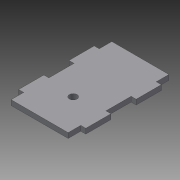
# Autodesk Inventor part: top
Saved by Autodesk Inventor 2015 (Build 190159000, 159)
## iProperties
Created: 2017-03-04
Part Number: top
Material: Generic
Document SubType Name: Modeling
Designer: Guy
Density: 1 g/cm^3
Appearance: Default
Author: Guy
Autodesk Inventor part; units mm, degrees
ref_plane "YZ Plane" through (0, 0, 0) normal (1, 0, 0) x (0, 1, 0)
ref_plane "XZ Plane" through (0, 0, 0) normal (0, 1, 0) x (-1, 0, 0)
ref_plane "XY Plane" through (0, 0, 0) normal (0, 0, 1) x (1, 0, 0)
sketch "Sketch1" plane through (0, 0, 0) normal (0, 0, 1) x (1, 0, 0)
  line L0 (0, 0) -> (120, 0)
  line L1 (120, 0) -> (120, 80)
  line L2 (120, 80) -> (0, 80)
  line L3 (0, 80) -> (0, 0)
  dimension "d0" = 120
  dimension "d1" = 80
  constraints: 8 end point, 2 parallel, 1 horizontal, 1 perpendicular
  measures "d0" distance of L2.end L1.end
  measures "d1" distance of L1.end L0.end
extrude "Extrusion1" add sketch "Sketch1" along normal blind 6
sketch "Sketch2" plane through (0, 0, 6) normal (0, 0, 1) x (1, 0, 0)
  line L0 (0, 0) -> (120, 0) projected
  line L1 (120, 0) -> (120, 80) projected
  line L2 (120, 80) -> (0, 80) projected
  line L3 (0, 80) -> (0, 0) projected
  line L4 (0, 80) -> (15, 80)
  line L5 (15, 80) -> (15, 74)
  line L6 (15, 74) -> (0, 74)
  line L7 (0, 74) -> (0, 80)
  line L8 (120, 80) -> (0, 80) projected
  line L9 (45, 80) -> (75, 80)
  line L10 (75, 80) -> (75, 74)
  line L11 (75, 74) -> (45, 74)
  line L12 (45, 74) -> (45, 80)
  line L13 (120, 80) -> (105, 80)
  line L14 (105, 80) -> (105, 74)
  line L15 (105, 74) -> (120, 74)
  line L16 (120, 74) -> (120, 80)
  line L17 (120, 0) -> (105, 0)
  line L18 (105, 0) -> (105, 6)
  line L19 (105, 6) -> (120, 6)
  line L20 (120, 6) -> (120, 0)
  line L21 (0, 0) -> (120, 0) projected
  line L22 (75, 0) -> (45, 0)
  line L23 (45, 0) -> (45, 6)
  line L24 (45, 6) -> (75, 6)
  line L25 (75, 6) -> (75, 0)
  line L26 (0, 0) -> (15, 0)
  line L27 (15, 0) -> (15, 6)
  line L28 (15, 6) -> (0, 6)
  line L29 (0, 6) -> (0, 0)
  dimension "d4" = 6
  dimension "d5" = 6
  dimension "d6" = 15
  dimension "d7" = 30
  dimension "d8" = 30
  dimension "d9" = 15
  constraints: 48 end point, 12 parallel, 7 point on line, 6 horizontal, 6 perpendicular, 3 collinear
  measures "d4" distance between parallel lines of L2 L6
  measures "d5" distance between parallel lines of L26 L28
  measures "d6" distance between parallel lines of L3 L5
  measures "d7" distance between parallel lines of L10 L12
  measures "d8" distance between parallel lines of L5 L12
  measures "d9" distance between parallel lines of L1 L14
extrude "Extrusion2" cut sketch "Sketch2" against normal up to next contours L3 L28 L27 L0 | L23 L24 L25 L0 | L3 L2 L5 L6 | L18 L19 L1 L0 | L2 L10 L11 L12 | L15 L14 L2 L1
sketch "Sketch4" plane through (0, 0, 6) normal (0, 0, 1) x (1, 0, 0)
  circle A0 centre (40, 40) radius 4.6
  line L0 (0, 74) -> (0, 6) projected
  line L1 (45, 80) -> (15, 80) projected
  point P0 (0, 0)
  dimension "d14" = 40
  dimension "d15" = 40
  dimension "d16" = 9.2
  constraints: 1 centre point
  measures "d14" distance from line of L0 A0.centre
  measures "d15" distance from line of A0.centre L1
  measures "d16" diameter of A0
extrude "Extrusion4" cut sketch "Sketch4" against normal up to next
body "Solid1"
